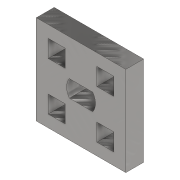
# Autodesk Inventor part: motor_bottom
Saved by Autodesk Inventor 2020 (Build 240168000, 168)
## iProperties
Created: 2021-05-10
Part Number: motor_bottom
Material: Generic
Document SubType Name: Modeling
Designer: Hsu Daniel
Density: 1 g/cm^3
Appearance: Diamond Plate
Author: Hsu Daniel
Autodesk Inventor part; units mm, degrees
ref_plane "YZ Plane" through (0, 0, 0) normal (1, 0, 0) x (0, 1, 0)
ref_plane "XZ Plane" through (0, 0, 0) normal (0, 1, 0) x (-1, 0, 0)
ref_plane "XY Plane" through (0, 0, 0) normal (0, 0, 1) x (1, 0, 0)
sketch "Sketch1" plane through (0, 0, 0) normal (0, 0, 1) x (1, 0, 0)
  line L0 (-1.96, -1.4194) -> (1.96, -1.4194)
  line L1 (1.96, 1.4194) -> (-1.96, 1.4194)
  arc A0 (-1.96, 1.4194) -> (-1.96, -1.4194) centre (0, 0) ccw
  arc A1 (1.96, -1.4194) -> (1.96, 1.4194) centre (0, 0) ccw
  line L2 (-7.5, -7.5) -> (7.5, -7.5)
  line L3 (7.5, -7.5) -> (7.5, 7.5)
  line L4 (7.5, 7.5) -> (-7.5, 7.5)
  line L5 (-7.5, 7.5) -> (-7.5, -7.5)
  line L6 (-7.5, -7.5) -> (7.5, 7.5) construction
  line L7 (7.5, -7.5) -> (-7.5, 7.5) construction
  line L8 (-5.5, 2.58) -> (-2.66, 2.58)
  line L9 (-2.66, 2.58) -> (-2.66, 5.5)
  line L10 (-2.66, 5.5) -> (-5.5, 5.5)
  line L11 (-5.5, 5.5) -> (-5.5, 2.58)
  line L12 (0, 0) -> (0, 4.08) construction
  line L13 (0, 0) -> (5.4269, 0) construction
  line L14 (5.5, 2.58) -> (2.66, 2.58)
  line L15 (2.66, 2.58) -> (2.66, 5.5)
  line L16 (2.66, 5.5) -> (5.5, 5.5)
  line L17 (5.5, 5.5) -> (5.5, 2.58)
  line L18 (-5.5, -2.58) -> (-2.66, -2.58)
  line L19 (-2.66, -2.58) -> (-2.66, -5.5)
  line L20 (-2.66, -5.5) -> (-5.5, -5.5)
  line L21 (-5.5, -5.5) -> (-5.5, -2.58)
  line L22 (2.66, -2.58) -> (2.66, -5.5)
  line L23 (2.66, -5.5) -> (5.5, -5.5)
  line L24 (5.5, -5.5) -> (5.5, -2.58)
  line L25 (5.5, -2.58) -> (2.66, -2.58)
  point P0 (0, -4.08)
  dimension "d3" = 3.92
  dimension "d4" = 2.42
  dimension "d5" = 15
  dimension "d7" = 2.84
  dimension "d8" = 2.92
  dimension "d9" = 2
  dimension "d10" = 2
  constraints: 52 end point, 13 symmetric about line, 5 parallel, 4 horizontal, 4 point on circle, 2 centre point, 2 equal length, 2 midpoint, 2 perpendicular, 1 coincident, 1 concentric, 1 vertical
  measures "d3" distance of L1.start L1.end
  measures "d4" radius of A1
  measures "d5" distance of L4.end L3.end
  measures "d7" distance of L10.end L9.end
  measures "d8" distance of L8.end L9.end
  measures "d9" distance between parallel lines of L4 L10
  measures "d10" distance between parallel lines of L5 L11
extrude "Extrusion1" add sketch "Sketch1" along normal blind 3
body "Solid1"
